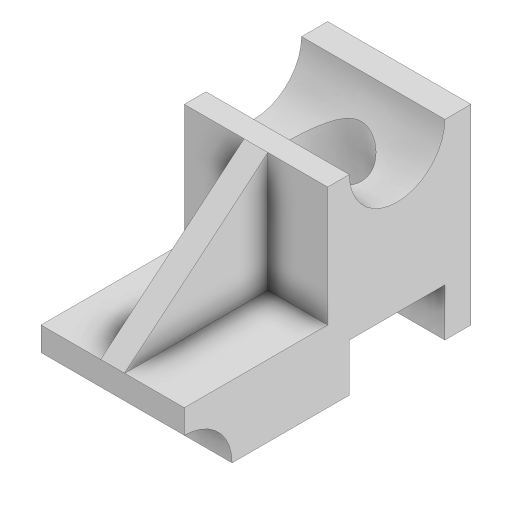
# Autodesk Inventor part: Корпус
Saved by Autodesk Inventor 2023.2 (Build 272271030, 271C)
## iProperties
Created: 2023-10-13
Part Number: Корпус
Material: Типовые
Document SubType Name: Modeling
Designer: User
Density: 1 g/cm^3
Appearance: По умолчанию
Author: User
Autodesk Inventor part; units mm, degrees
ref_plane "YZ Plane" through (0, 0, 0) normal (1, 0, 0) x (0, 1, 0)
ref_plane "XZ Plane" through (0, 0, 0) normal (0, 1, 0) x (-1, 0, 0)
ref_plane "XY Plane" through (0, 0, 0) normal (0, 0, 1) x (1, 0, 0)
sketch "Эскиз1" plane through (0, 0, 0) normal (1, 0, 0) x (0, 1, 0)
  line L0 (0, -30.9291) -> (80, -30.9291)
  line L1 (80, 29.0709) -> (30, 29.0709)
  line L2 (30, 29.0709) -> (30, 89.0709)
  line L3 (30, 89.0709) -> (20, 89.0709)
  line L4 (80, 29.0709) -> (30, 89.0709)
  arc A0 (0, 69.0709) -> (20, 89.0709) centre (0, 89.0709) ccw
  arc A1 (80, 20) -> (80, -20) centre (80, 0) ccw
  line L5 (0, 20) -> (20, 20)
  line L6 (20, 20) -> (20, -20)
  line L7 (20, -20) -> (0, -20)
  line L8 (0, -20) -> (0, -30.9291)
  line L9 (80, -30.9291) -> (80, -20)
  line L10 (80, 20) -> (80, 29.0709)
  line L11 (0, 69.0709) -> (0, 20)
  point P0 (0, 0)
  constraints: 24 end point, 9 perpendicular, 4 point on circle, 2 centre point, 2 vertical, 1 horizontal, 1 parallel
extrude "Выдавливание1" add sketch "Эскиз1" along normal mid plane 60 contours L8 L7 L6 L5 L11 A0 L3 L2 L1 L10 A1 L9 L0
extrude "Выдавливание2" add sketch "Эскиз1" along normal mid plane 10 contours L1 L2 L4
sketch "Эскиз3" plane through (0, 0, 0) normal (0, 1, 0) x (-1, 0, 0)
  circle A0 centre (0, 0) radius 15
  dimension "d12" = 30
  constraints: 1 centre point, 1 coincident
  measures "d12" diameter of A0
extrude "Выдавливание3" cut sketch "Эскиз3" along normal blind 100
